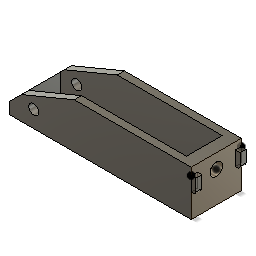
PS-Extra-Bracket (Autodesk Fusion 360 design; units mm, degrees)
Autodesk Fusion 360 part; units mm, degrees
sketch "Sketch1" plane through (0, 0, 0) normal (0, 1, 0) x (1, 0, 0)
  line L0 (0, 0) -> (70, 0)
  line L1 (70, 0) -> (70, -15)
  line L2 (70, -15) -> (0, -15)
  line L3 (0, -15) -> (0, 0)
  line L4 (-3, 3) -> (73, 3)
  line L5 (73, 3) -> (73, -18)
  line L6 (73, -18) -> (-3, -18)
  line L7 (-3, -18) -> (-3, 3)
  line L8 (68, 0) -> (68, -15)
  line L9 (12.5, 0) -> (12.5, -15)
  dimension "d1" = 70
  dimension "d2" = 15
  dimension "d3" = 3
  dimension "d6" = 2
  dimension "d27" = 12.5
  measures "d1" distance of L0.start L0.end
  measures "d2" distance of L0.start L2.end
  measures "d6" distance of L1 L8
  measures "d27" distance of L3 L9
extrude "Extrude1" add sketch "Sketch1" against normal blind 3 contours L0 L2 L8 L9 | L0 L1 L2 L8 | L4 L5 L6 L7
extrude "Extrude2" add sketch "Sketch1" along normal blind 16 contours L0 L1 L2 L8 | L4 L5 L6 L7
sketch "Sketch2" plane through (73, 0, 0) normal (1, 0, 0) x (0, 0, -1)
  line L0 (-18, 16) -> (-18, -3)
  line L1 (-18, -3) -> (3, -3)
  line L2 (3, -3) -> (3, 16)
  line L3 (3, 16) -> (-18, 16)
  circle A0 centre (-7.5, 10) radius 2.6
  line L4 (3, 13) -> (0.5, 13)
  line L5 (0.5, 13) -> (0.5, 7)
  line L6 (0.5, 7) -> (3, 7)
  line L7 (3, 7) -> (3, 13)
  line L8 (-18, 13) -> (-15.5, 13)
  line L9 (-15.5, 13) -> (-15.5, 7)
  line L10 (-15.5, 7) -> (-18, 7)
  line L11 (-18, 7) -> (-18, 13)
  dimension "d9" = 5.2
  dimension "d10" = 10.5
  dimension "d11" = 2.5
  dimension "d12" = 6
  dimension "d13" = 2.5
  dimension "d14" = 6
  dimension "d15" = 3
  dimension "d16" = 3
  dimension "d17" = 6
  measures "d9" diameter of A0
  measures "d10" distance of L0 A0.centre
  measures "d11" distance of L4.start L4.end
  measures "d12" distance of L4.start L6.end
  measures "d13" distance of L8.start L8.end
  measures "d14" distance of L8.start L10.end
  measures "d15" distance of L3 L4
  measures "d16" distance of L3 L8
  measures "d17" distance of L3 A0.centre
extrude "Extrude3" add sketch "Sketch2" along normal blind 2 contours L0 L8 L9 L10 L11 | L2 L4 L5 L6 L7
extrude "Extrude4" cut sketch "Sketch2" against normal blind 5 contours A0
sketch "Sketch3" plane through (0, 0, -3) normal (0, 0, -1) x (-1, 0, 0)
  line L0 (-73, 7) -> (-73, -3)
  line L1 (-73, -3) -> (3, -3)
  line L2 (3, -3) -> (3, 16)
  line L3 (3, 16) -> (-73, 16)
  line L4 (-73, 16) -> (-73, 13)
  line L5 (-73, 13) -> (-75, 13)
  line L6 (-75, 13) -> (-75, 7)
  line L7 (-75, 7) -> (-73, 7)
  circle A0 centre (-7, 4) radius 2.1
  dimension "d22" = 4.2
  dimension "d23" = 12
  dimension "d24" = 10
  measures "d22" diameter of A0
  measures "d23" distance of L3 A0.centre
  measures "d24" distance of L2 A0.centre
extrude "Extrude5" cut sketch "Sketch3" against normal blind 21 contours A0
fillet "Fillet1" radius 1 2 edges at (75, 7, 16.75) (75, 7, -1.75)
chamfer "Chamfer3" distance 14 angle 45 1 edges at (-3, 16, 7.5)
chamfer "Chamfer4" distance 13 angle 45 2 edges at (11, 16, 16.5) (11, 16, -1.5)
equation "d10 = ( 21 / 2 ) * 1 mm"
